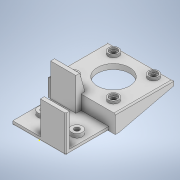
# Autodesk Inventor part: stepperBracketVertical
Saved by Autodesk Inventor 2020 (Build 240168000, 168)
## iProperties
Created: 2020-01-08
Part Number: stepperBracketVertical
Material: Generic
Document SubType Name: Modeling
Designer: PAB
Density: 1 g/cm^3
Appearance: Default
Author: PAB
Autodesk Inventor part; units mm, degrees
ref_plane "YZ Plane" through (0, 0, 0) normal (1, 0, 0) x (0, 1, 0)
ref_plane "XZ Plane" through (0, 0, 0) normal (0, 1, 0) x (-1, 0, 0)
ref_plane "XY Plane" through (0, 0, 0) normal (0, 0, 1) x (1, 0, 0)
sketch "Sketch1" plane through (0, 0, 0) normal (0, 1, 0) x (-1, 0, 0)
  line L0 (20.5, 16.2) -> (-20.5, 16.2)
  line L1 (-20.5, 16.2) -> (-20.5, -16.2)
  line L2 (-20.5, -16.2) -> (20.5, -16.2)
  line L3 (20.5, -16.2) -> (20.5, 16.2)
  point P0 (0, 0)
  dimension "d0" = 41
  dimension "d1" = 32.4
  constraints: 8 end point, 2 parallel, 1 horizontal, 1 perpendicular
  measures "d0" distance of L2.end L1.end
  measures "d1" distance of L1.end L0.end
extrude "Extrusion1" add sketch "Sketch1" along normal blind 3
sketch "Sketch3" plane through (0, 3, 0) normal (0, 1, 0) x (1, 0, 0)
  line L0 (-20.5, -16.2) -> (20.5, -16.2) projected
  line L1 (-20.5, 16.2) -> (-20.5, -16.2) projected
  line L2 (20.5, -16.2) -> (-20.5, -16.2)
  line L3 (-20.5, -16.2) -> (-20.5, -13.2)
  line L4 (-20.5, -13.2) -> (20.5, -13.2)
  line L5 (20.5, -13.2) -> (20.5, -16.2)
  line L6 (20.5, 16.2) -> (-20.5, 16.2) projected
  line L7 (20.5, 16.2) -> (-20.5, 16.2)
  line L8 (-20.5, 16.2) -> (-20.5, 13.2)
  line L9 (-20.5, 13.2) -> (20.5, 13.2)
  line L10 (20.5, 13.2) -> (20.5, 16.2)
  point P0 (0, 0)
  dimension "d8" = 3
  dimension "d9" = 3
  constraints: 16 end point, 4 parallel, 2 horizontal, 2 perpendicular, 2 point on line
  measures "d8" distance of L2.end L3.end
  measures "d9" distance of L8.end L7.end
extrude "Extrusion3" add sketch "Sketch3" along normal blind 25.4
sketch "Sketch4" plane through (20.5, 0, -16.2) normal (0, 0, -1) x (-1, 0, 0)
  line L0 (41, 3) -> (0, 3) projected
  line L1 (0, 28.4) -> (41, 28.4) projected
  line L2 (0, 3) -> (21.5, 3)
  line L3 (21.5, 3) -> (21.5, 28.4)
  line L4 (21.5, 28.4) -> (0, 28.4)
  line L5 (0, 28.4) -> (0, 3)
  point P0 (20.5, 0)
  dimension "d12" = 21.5
  constraints: 8 end point, 2 parallel, 1 horizontal, 1 perpendicular, 1 point on line
  measures "d12" distance of L4.end L3.end
extrude "Extrusion4" cut sketch "Sketch4" against normal blind 3
sketch "Sketch5" plane through (-20.5, 0, 16.2) normal (0, 0, 1) x (1, 0, 0)
  line L0 (41, 28.4) -> (0, 28.4) projected
  line L1 (19.5, 3) -> (41, 3) projected
  line L2 (0, 28.4) -> (21.5, 28.4)
  line L3 (21.5, 28.4) -> (21.5, 3)
  line L4 (21.5, 3) -> (0, 3)
  line L5 (0, 3) -> (0, 28.4)
  point P0 (20.5, 0)
  dimension "d15" = 21.5
  constraints: 8 end point, 2 parallel, 1 horizontal, 1 perpendicular, 1 point on line
  measures "d15" distance of L3.end L4.end
extrude "Extrusion5" cut sketch "Sketch5" against normal blind 3
sketch "Sketch6" plane through (0, 3, 0) normal (0, 1, 0) x (1, 0, 0)
  circle A0 centre (13, 0) radius 4.25
  circle A1 centre (-13, 0) radius 4.25
  line L0 (20.5, -13.2) -> (20.5, 16.2) projected
  line L1 (-20.5, 13.2) -> (-20.5, -16.2) projected
  point P0 (0, 0)
  dimension "d20" = 8.5
  dimension "d21" = 8.5
  dimension "d54" = 7.5
  dimension "d65" = 26
  dimension "d66" = 7.5
  constraints: 2 centre point
  measures "d20" diameter of A0
  measures "d21" diameter of A1
  measures "d54" distance from line of L1 A1.centre
  measures "d65" distance of A0.centre A1.centre
  measures "d66" distance from line of L0 A0.centre
extrude "Extrusion6" add sketch "Sketch6" along normal blind 3
sketch "Sketch7" plane through (0, 0, 0) normal (0, -1, 0) x (1, 0, 0)
  circle A0 centre (-13, 0) radius 4.25 projected
  circle A1 centre (-13, 0) radius 2
  circle A2 centre (13, 0) radius 4.25 projected
  circle A3 centre (13, 0) radius 2
  point P0 (0, 0)
  dimension "d24" = 4
  dimension "d25" = 4
  constraints: 2 centre point, 2 coincident
  measures "d24" diameter of A1
  measures "d25" diameter of A3
extrude "Extrusion7" cut sketch "Sketch7" against normal blind 6 contours A1 | A3
sketch "Sketch8" plane through (0, 0, 0) normal (0, -1, 0) x (1, 0, 0)
  circle A0 centre (-13, 0) radius 2 projected
  circle A1 centre (-13, 0) radius 3
  circle A2 centre (13, 0) radius 2 projected
  circle A3 centre (13, 0) radius 3
  point P0 (0, 0)
  dimension "d28" = 6
  dimension "d29" = 6
  constraints: 2 centre point, 2 coincident
  measures "d28" diameter of A1
  measures "d29" diameter of A3
extrude "Extrusion8" cut sketch "Sketch8" against normal blind 3 contours A0 | A1 | A2 | A3
sketch "Sketch14" plane through (-20.5, 0, 16.2) normal (0, 0, 1) x (1, 0, 0)
  point P0 (20.5, 0)
sketch "Sketch15" plane through (20.5, 0, -16.2) normal (0, 0, -1) x (-1, 0, 0)
  line L0 (0, 0) -> (0, 3) projected
  line L1 (41, 0) -> (41, 28.4) projected
  line L2 (0, 0) -> (41, 0)
  line L3 (41, 0) -> (41, 14)
  line L4 (41, 14) -> (0, 14)
  line L5 (0, 14) -> (0, 0)
  line L6 (21.5, 28.4) -> (41, 28.4) projected
  line L7 (41, 14) -> (37, 14)
  line L8 (37, 14) -> (37, 28.4)
  line L9 (37, 28.4) -> (41, 28.4)
  line L10 (41, 28.4) -> (41, 14)
  line L11 (21.5, 3) -> (21.5, 28.4) projected
  line L12 (21.5, 14) -> (25.5, 14)
  line L13 (25.5, 14) -> (25.5, 28.4)
  line L14 (25.5, 28.4) -> (21.5, 28.4)
  line L15 (21.5, 28.4) -> (21.5, 14)
  point P0 (20.5, 0)
  dimension "d67" = 14
  dimension "d68" = 4
  dimension "d69" = 4
  constraints: 24 end point, 6 parallel, 5 point on line, 3 horizontal, 3 perpendicular
  measures "d67" distance of L3.end L2.end
  measures "d68" distance of L8.end L9.end
  measures "d69" distance of L14.end L13.end
extrude "Extrusion14" add sketch "Sketch15" along normal blind 4 contours L0 L5 L4 L1 L2 | L4 L8 L6 L1 | L11 L6 L13 L4
sketch "Sketch16" plane through (20.5, 0, -20.2) normal (0, 0, -1) x (-1, 0, 0)
  line L0 (21.5, 14) -> (0, 14) projected
  line L1 (41, 3) -> (41, 28.4) projected
  line L2 (0, 14) -> (41, 14)
  line L3 (41, 14) -> (41, 10)
  line L4 (41, 10) -> (0, 10)
  line L5 (0, 10) -> (0, 14)
  point P0 (20.5, 0)
  point P1 (41, 14)
  dimension "d72" = 4
  constraints: 8 end point, 2 parallel, 1 horizontal, 1 perpendicular, 1 point on line
  measures "d72" distance of L2.end L3.end
extrude "Extrusion15" add sketch "Sketch16" along normal blind 42.3
sketch "Sketch17" plane through (-1, 14, -16.2) normal (0, 1, 0) x (1, 0, 0)
  circle A0 centre (16.5, 40.65) radius 4
  circle A1 centre (-14.5, 40.65) radius 4
  circle A2 centre (-14.5, 9.65) radius 4
  circle A3 centre (16.5, 9.65) radius 4
  point P0 (1, -16.2)
  dimension "d76" = 8
  dimension "d77" = 8
  dimension "d78" = 8
  dimension "d79" = 8
  constraints: 4 centre point
  measures "d76" diameter of A0
  measures "d77" diameter of A1
  measures "d78" diameter of A2
  measures "d79" diameter of A3
extrude "Extrusion16" add sketch "Sketch17" along normal blind 2
sketch "Sketch18" plane through (-1, 14, -16.2) normal (0, 1, 0) x (1, 0, 0)
  circle A0 centre (1, 25.15) radius 12.5
  circle A1 centre (-14.5, 40.65) radius 4 projected
  circle A2 centre (-14.5, 40.65) radius 2
  circle A3 centre (-14.5, 9.65) radius 4 projected
  circle A4 centre (-14.5, 9.65) radius 2
  circle A5 centre (16.5, 9.65) radius 4 projected
  circle A6 centre (16.5, 9.65) radius 2
  circle A7 centre (16.5, 40.65) radius 4 projected
  circle A8 centre (16.5, 40.65) radius 2
  point P0 (1, -16.2)
  dimension "d82" = 25
  dimension "d83" = 4
  dimension "d84" = 4
  dimension "d85" = 4
  dimension "d86" = 4
  constraints: 5 centre point, 4 coincident
  measures "d82" diameter of A0
  measures "d83" diameter of A2
  measures "d84" diameter of A4
  measures "d85" diameter of A6
  measures "d86" diameter of A8
extrude "Extrusion17" cut sketch "Sketch18" along normal mid plane 10 contours A0 | A2 | A4 | A6 | A8
sketch "Sketch19" plane through (15.5, 16, -25.85) normal (0, 1, 0) x (1, 0, 0)
  circle A0 centre (-31, 0) radius 2 projected
  circle A1 centre (-31, 0) radius 3
  circle A2 centre (0, 0) radius 2 projected
  circle A3 centre (0, 0) radius 3
  circle A4 centre (0, 31) radius 2 projected
  circle A5 centre (0, 31) radius 3
  circle A6 centre (-31, 31) radius 2 projected
  circle A7 centre (-31, 31) radius 3
  point P0 (-15.5, -25.85)
  dimension "d89" = 6
  dimension "d90" = 6
  dimension "d91" = 6
  dimension "d92" = 6
  constraints: 4 centre point, 4 coincident
  measures "d89" diameter of A1
  measures "d90" diameter of A3
  measures "d91" diameter of A5
  measures "d92" diameter of A7
extrude "Extrusion18" cut sketch "Sketch19" against normal blind 1.5 contours A0 | A1 | A2 | A3 | A4 | A5 | A6 | A7
sketch "Sketch20" plane through (20.5, 0, 16.2) normal (1, 0, 0) x (0, 0, -1)
  line L0 (36.4, 14) -> (78.7, 14) projected
  line L1 (78.7, 14) -> (36.4, 14)
  line L2 (36.4, 14) -> (36.4, 10)
  line L3 (36.4, 10) -> (78.7, 10)
  line L4 (78.7, 10) -> (78.7, 14)
  line L5 (32.4, 14) -> (32.4, 3) projected
  line L6 (36.4, 0) -> (36.4, 10) projected
  line L7 (32.4, 14) -> (36.4, 14)
  line L8 (36.4, 14) -> (36.4, 0)
  line L9 (36.4, 0) -> (32.4, 0)
  line L10 (32.4, 0) -> (32.4, 14)
  point P0 (16.2, 0)
  constraints: 16 end point, 4 parallel, 2 horizontal, 2 perpendicular
extrude "Extrusion19" add sketch "Sketch20" along normal blind 5
sketch "Sketch21" plane through (-20.5, 0, 16.2) normal (-1, 0, 0) x (0, 0, 1)
  line L0 (-78.7, 14) -> (-32.4, 14) projected
  line L1 (-36.4, 10) -> (-78.7, 10) projected
  line L2 (-78.7, 14) -> (-36.4, 14)
  line L3 (-36.4, 14) -> (-36.4, 10)
  line L4 (-36.4, 10) -> (-78.7, 10)
  line L5 (-78.7, 10) -> (-78.7, 14)
  line L6 (0, 0) -> (-36.4, 0) projected
  line L7 (-32.4, 0) -> (-36.4, 0)
  line L8 (-36.4, 0) -> (-36.4, 14)
  line L9 (-36.4, 14) -> (-32.4, 14)
  line L10 (-32.4, 14) -> (-32.4, 0)
  point P0 (-16.2, 0)
  constraints: 16 end point, 4 parallel, 2 horizontal, 2 perpendicular, 1 point on line
extrude "Extrusion20" add sketch "Sketch21" along normal blind 5
sketch "Sketch22" plane through (25.5, 10, -62.5) normal (0, -1, 0) x (1, 0, 0)
  line L0 (0, 0) -> (0, 46.3) projected
  line L1 (-51, 42.3) -> (0, 42.3) projected
  line L2 (0, 0) -> (-4, 0)
  line L3 (-4, 0) -> (-4, 42.3)
  line L4 (-4, 42.3) -> (0, 42.3)
  line L5 (0, 42.3) -> (0, 0)
  line L6 (-51, 46.3) -> (-51, 0) projected
  line L7 (-51, 0) -> (-47, 0)
  line L8 (-47, 0) -> (-47, 42.3)
  line L9 (-47, 42.3) -> (-51, 42.3)
  line L10 (-51, 42.3) -> (-51, 0)
  point P0 (-25.5, 62.5)
  dimension "d99" = 4
  dimension "d100" = 4
  constraints: 16 end point, 4 parallel, 2 horizontal, 2 perpendicular, 2 point on line
  measures "d99" distance of L3.end L4.end
  measures "d100" distance of L9.end L8.end
extrude "Extrusion21" add sketch "Sketch22" along normal blind 10
sketch "Sketch23" plane through (25.5, 0, 16.2) normal (1, 0, 0) x (0, 0, -1)
  line L0 (36.4, 10) -> (78.7, 10) projected
  line L1 (36.4, 10) -> (36.4, 0) projected
  line L2 (78.7, 10) -> (36.4, 0)
  line L3 (36.4, 0) -> (78.7, 0)
  line L4 (78.7, 0) -> (78.7, 10)
  point P0 (16.2, 0)
  constraints: 6 end point, 2 perpendicular
extrude "Extrusion22" cut sketch "Sketch23" against normal blind 60 contours L4 L3 L2
sketch "Sketch24" plane through (-1, 3, -13.2) normal (1, 0, 0) x (0, 0, -1)
  line L0 (7, 25.4) -> (7, 11) projected
  line L1 (3, 25.4) -> (3, 11) projected
  line L2 (7, 11) -> (3, 25.4)
  line L3 (0, 25.4) -> (7, 25.4) projected
  line L4 (3, 25.4) -> (7, 25.4)
  line L5 (7, 25.4) -> (7, 11)
  point P0 (-13.2, -3)
  constraints: 6 end point, 1 collinear, 1 perpendicular
extrude "Extrusion23" cut sketch "Sketch24" against normal blind 60
sketch "Sketch25" plane through (25.5, 0, 16.2) normal (1, 0, 0) x (0, 0, -1)
  line L0 (32.4, 14) -> (32.4, 28.4) projected
  line L1 (32.4, 14) -> (33.4, 14)
  line L2 (33.4, 14) -> (33.4, 3)
  line L3 (33.4, 3) -> (32.4, 3)
  line L4 (32.4, 3) -> (32.4, 14)
  point P0 (16.2, 0)
  dimension "d107" = 1
  constraints: 8 end point, 2 parallel, 1 horizontal, 1 perpendicular
  measures "d107" distance of L2.end L3.end
extrude "Extrusion24" cut sketch "Sketch25" against normal blind 26.5
sketch "Sketch26" plane through (25.5, 0, 16.2) normal (1, 0, 0) x (0, 0, -1)
  line L0 (33.4, 3) -> (32.4, 3) projected
  line L1 (32.4, 0) -> (36.4, 0) projected
  line L2 (32.4, 3) -> (33.4, 3)
  line L3 (33.4, 3) -> (33.4, 0)
  line L4 (33.4, 0) -> (32.4, 0)
  line L5 (32.4, 0) -> (32.4, 3)
  point P0 (16.2, 0)
  dimension "d110" = 1
  constraints: 8 end point, 2 parallel, 1 horizontal, 1 perpendicular, 1 point on line
  measures "d110" distance of L3.end L4.end
extrude "Extrusion25" cut sketch "Sketch26" against normal blind 5
fillet "Fillet2" radius 1 7 edges at (20.5, 14.2, 16.2) (20.5, 0, -0.5) (0, 0, 16.2) (-20.5, 0, 0) (-25.5, 14, -39.35) (0, 14, -62.5) (25.5, 14, -39.85)
body "Solid1"
